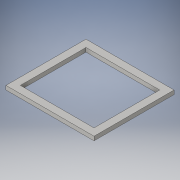
# Autodesk Inventor part: BAck_chasis
Saved by Autodesk Inventor 2016 (Build 200138000, 138)
## iProperties
Created: 2016-02-28
Part Number: BAck_chasis
Material: Generic
Document SubType Name: Modeling
Designer: torti_000
Density: 1 g/cm^3
Appearance: Default
Author: torti_000
Autodesk Inventor part; units mm, degrees
ref_plane "YZ Plane" through (0, 0, 0) normal (1, 0, 0) x (0, 1, 0)
ref_plane "XZ Plane" through (0, 0, 0) normal (0, 1, 0) x (-1, 0, 0)
ref_plane "XY Plane" through (0, 0, 0) normal (0, 0, 1) x (1, 0, 0)
sketch "Sketch1" plane through (0, 0, 0) normal (0, 1, 0) x (-1, 0, 0)
  line L0 (0, 0) -> (139.7, 0)
  line L1 (139.7, 0) -> (139.7, -127)
  line L2 (139.7, -127) -> (0, -127)
  line L3 (0, -127) -> (0, 0)
  line L4 (128.27, -115.57) -> (128.27, -11.43)
  line L5 (128.27, -11.43) -> (11.43, -11.43)
  line L6 (11.43, -11.43) -> (11.43, -115.57)
  line L7 (11.43, -115.57) -> (128.27, -115.57)
  dimension "d0" = 139.7
  dimension "d1" = 127
  dimension "d2" = 11.43
  constraints: 16 end point, 6 perpendicular, 1 horizontal, 3 other
  measures "d0" distance of L0.start L0.end
  measures "d1" distance of L0.end L1.end
  measures "d2" distance between parallel lines of L1 L4
extrude "Extrusion1" add sketch "Sketch1" along normal blind 6.35
body "Solid1"
